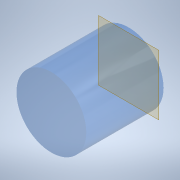
# Autodesk Inventor part: wodaxD
Saved by Autodesk Inventor 2021 (Build 250183000, 183)
## iProperties
Created: 2021-05-23
Part Number: wodaxD
Material: Woda
Document SubType Name: Modeling
Designer: Wojciech Wołczek
Density: 0.9983 g/cm^3
Appearance: Tropikalnie niebieska
Author: Wojciech Wołczek
Autodesk Inventor part; units mm, degrees
ref_plane "YZ Plane" through (0, 0, 0) normal (1, 0, 0) x (0, 1, 0)
ref_plane "XZ Plane" through (0, 0, 0) normal (0, 1, 0) x (-1, 0, 0)
ref_plane "XY Plane" through (0, 0, 0) normal (0, 0, 1) x (1, 0, 0)
ref_plane "Płaszczyzna konstrukcyjna1" through (0, 0, 0) normal (0, 0, 1) x (1, 0, 0)
sketch "Szkic1" plane through (0, 0, 0) normal (0, 0, 1) x (1, 0, 0)
  circle A0 centre (110, 0) radius 110 projected
  circle A1 centre (110, 0) radius 140 projected
  point P0 (0, 0)
  constraints: 1 horizontal alignment
extrude "Wyciągnięcie proste1" add sketch "Szkic1" along normal blind 310 contours A0 | A1
fillet "Zaokrąglenie1" radius 30 1 edges at (-30, 0, 0)
sketch "Szkic2" plane through (110, 0, 310) normal (0, 0, 1) x (1, 0, 0)
  circle A0 centre (0, 0) radius 80
  circle A1 centre (0, 0) radius 140
  point P0 (-110, 0)
  dimension "d3" = 160
  constraints: 2 centre point, 1 coincident
  measures "d3" diameter of A0
extrude "Wyciągnięcie proste2" cut sketch "Szkic2" against normal blind 30
fillet "Zaokrąglenie2" radius 30 1 edges at (-30, 0, 280)
fillet "Zaokrąglenie3" radius 20 1 edges at (30, 0, 280)
sketch "Szkic3" plane through (110, 0, 310) normal (0, 0, 1) x (1, 0, 0)
  circle A0 centre (0, 0) radius 31.5
  point P0 (-110, 0)
  dimension "d8" = 63
  constraints: 1 centre point
  measures "d8" diameter of A0
extrude "Wyciągnięcie proste3" cut sketch "Szkic3" against normal blind 123
